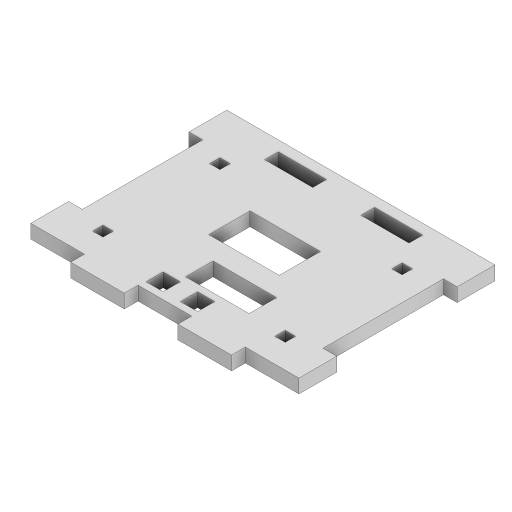
# Autodesk Inventor part: Front
Saved by Autodesk Inventor 2023.3 (Build 273359000, 359)
## iProperties
Created: 2024-06-25
Part Number: Front
Material: Generic
Document SubType Name: Modeling
Designer: David Zindović
Density: 1 g/cm^3
Appearance: Default
Author: David Zindović
Autodesk Inventor part; units mm, degrees
ref_plane "YZ Plane" through (0, 0, 0) normal (1, 0, 0) x (0, 1, 0)
ref_plane "XZ Plane" through (0, 0, 0) normal (0, 1, 0) x (-1, 0, 0)
ref_plane "XY Plane" through (0, 0, 0) normal (0, 0, 1) x (1, 0, 0)
sketch "Sketch1" plane through (0, 0, 0) normal (0, 1, 0) x (-1, 0, 0)
  line L0 (39, 23) -> (-39, 23)
  line L1 (-39, 23) -> (-39, -38)
  line L2 (-39, -38) -> (39, -38)
  line L3 (39, -38) -> (39, 23)
  line L4 (-7, -31) -> (-21, -31)
  line L5 (-21, -31) -> (-21, -35)
  line L6 (-21, -35) -> (-7, -35)
  line L7 (-7, -35) -> (-7, -31)
  line L8 (-39, 8) -> (-35, 8)
  line L9 (-35, 8) -> (-35, -27)
  line L10 (-35, -27) -> (-39, -27)
  line L11 (-39, -27) -> (-39, 8)
  line L12 (-7.8, 23) -> (-23.4, 23)
  line L13 (-23.4, 23) -> (-23.4, 19)
  line L14 (-23.4, 19) -> (-7.8, 19)
  line L15 (-7.8, 19) -> (-7.8, 23)
  line L16 (0, 0) -> (0, -17.5171)
  line L17 (7, -31) -> (21, -31)
  line L18 (21, -31) -> (21, -35)
  line L19 (21, -35) -> (7, -35)
  line L20 (7, -35) -> (7, -31)
  line L21 (39, 8) -> (35, 8)
  line L22 (35, 8) -> (35, -27)
  line L23 (35, -27) -> (39, -27)
  line L24 (23.4, 23) -> (23.4, 19)
  line L25 (23.4, 19) -> (7.8, 19)
  line L26 (7.8, 19) -> (7.8, 23)
  line L27 (-39, 19) -> (39, 19)
  point P0 (0, -38)
  point P1 (-39, -7.5)
  point P2 (-7, -33)
  point P3 (7, -33)
  point P4 (-7.8, 19)
  point P5 (-23.4, 19)
  point P6 (-39, -27)
  point P7 (39, -27)
  point P8 (39, 8)
  point P9 (23.4, 19)
  point P10 (7.8, 19)
  point P11 (35, -9.5)
  point P12 (-35, -9.5)
  dimension "d0" = 61
  dimension "d1" = 78
  dimension "d2" = 14
  dimension "d3" = 4
  dimension "d4" = 3
  dimension "d5" = 7
  dimension "d6" = 35
  dimension "d7" = 11
  dimension "d8" = 15.6
  dimension "d9" = 15.6
  dimension "d12" = 4
  dimension "d13" = 4
  dimension "d35" = 4
  constraints: 56 end point, 9 symmetric about line, 5 midpoint, 5 parallel, 4 horizontal, 4 horizontal alignment, 4 point on line, 3 perpendicular, 1 collinear, 1 vertical, 1 vertical alignment
  measures "d0" distance of L0.end L1.end
  measures "d1" distance of L1.end L2.end
  measures "d2" distance of L6.end L5.end
  measures "d3" distance of L5.end L4.end
  measures "d4" distance between parallel lines of L2 L6
  measures "d5" horizontal distance of L16.start point (-7, -33)
  measures "d6" distance of L8.end L9.end
  measures "d7" distance between parallel lines of L2 L10
  measures "d8" distance of L13.end L14.end
  measures "d9" distance between parallel lines of L1 L13
  measures "d12" distance of L9.end L10.end
  measures "d13" distance of L12.end L13.end
  measures "d35" distance of L22.end L23.end
extrude "Extrusion1" add sketch "Sketch1" along normal mid plane 4 contours L24 L25 L26 L0 | L3 L21 L22 L23 L2 L1 L10 L9 L8 L27 L14 L25 | L15 L14 L13 L0
sketch "Sketch2" plane through (0, 2, 0) normal (0, 1, 0) x (1, 0, 0)
  line L0 (35, 27) -> (39, 27) projected
  line L1 (35, 27) -> (15.5, 27) construction
  line L2 (15.5, -2) -> (-3, -2)
  line L3 (-3, -2) -> (-3, -10)
  line L4 (-3, -10) -> (15.5, -10)
  line L5 (15.5, -10) -> (15.5, -2)
  line L6 (21, 31) -> (7, 31) projected
  line L7 (7.5, -17) -> (2.5, -17)
  line L8 (2.5, -17) -> (2.5, -12)
  line L9 (2.5, -12) -> (7.5, -12)
  line L10 (7.5, -12) -> (7.5, -17)
  line L11 (0, 0) -> (0, -2.2371)
  line L12 (-7.5, -17) -> (-2.5, -17)
  line L13 (-2.5, -17) -> (-2.5, -12)
  line L14 (-2.5, -12) -> (-7.5, -12)
  line L15 (-7.5, -12) -> (-7.5, -17)
  line L16 (28, -12) -> (25, -12)
  line L17 (25, -12) -> (25, -9)
  line L18 (25, -9) -> (28, -9)
  line L19 (28, -9) -> (28, -12)
  line L20 (35, -8) -> (35, 27) projected
  line L21 (23.4, -19) -> (39, -19) projected
  line L22 (-28, -12) -> (-25, -12)
  line L23 (-25, -12) -> (-25, -9)
  line L24 (-25, -9) -> (-28, -9)
  line L25 (-28, -9) -> (-28, -12)
  line L26 (-10.25, 16) -> (10.25, 16)
  line L27 (10.25, 16) -> (10.25, 4)
  line L28 (10.25, 4) -> (-10.25, 4)
  line L29 (-10.25, 4) -> (-10.25, 16)
  line L30 (39, 38) -> (-39, 38) projected
  line L31 (7.8, -23) -> (23.4, -23) projected
  line L32 (28, 22) -> (25, 22)
  line L33 (25, 22) -> (25, 25)
  line L34 (25, 25) -> (28, 25)
  line L35 (28, 25) -> (28, 22)
  line L36 (-28, 22) -> (-25, 22)
  line L37 (-25, 22) -> (-25, 25)
  line L38 (-25, 25) -> (-28, 25)
  line L39 (-28, 25) -> (-28, 22)
  point P0 (14, 31)
  point P1 (5, -17)
  point P2 (-5, -17)
  point P3 (28, -10.5)
  point P4 (31.2, -19)
  point P5 (-28, -10.5)
  point P6 (0, 16)
  point P7 (0, 38)
  point P8 (26.5, 22)
  point P9 (26.5, -9)
  point P10 (-26.5, 22)
  dimension "d14" = 19.5
  dimension "d15" = 18.5
  dimension "d16" = 8
  dimension "d17" = 41
  dimension "d20" = 5
  dimension "d21" = 5
  dimension "d22" = 5
  dimension "d23" = 43
  dimension "d26" = 3
  dimension "d27" = 3
  dimension "d28" = 7
  dimension "d31" = 20.5
  dimension "d32" = 12
  dimension "d33" = 6
  dimension "d34" = 11
  dimension "d36" = 3
  dimension "d37" = 3
  dimension "d38" = 31
  constraints: 68 end point, 15 symmetric about line, 10 parallel, 8 midpoint, 6 horizontal, 5 perpendicular, 3 vertical alignment, 1 vertical
  measures "d14" distance of L0.start L1.end
  measures "d15" distance of L3.end L4.end
  measures "d16" distance of L2.end L3.end
  measures "d17" distance from line of point (14, 31) L4
  measures "d20" distance of L8.end L9.end
  measures "d21" distance of L7.end L8.end
  measures "d22" horizontal distance of L11.start point (5, -17)
  measures "d23" distance between parallel lines of L6 L9
  measures "d26" distance of L17.end L18.end
  measures "d27" distance of L16.end L17.end
  measures "d28" distance from line of L20 point (28, -10.5)
  measures "d31" distance of L27.end L28.end
  measures "d32" distance of L26.end L27.end
  measures "d33" distance between parallel lines of L28 L2
  measures "d34" distance between parallel lines of L16 L31
  measures "d36" distance of L33.end L34.end
  measures "d37" distance of L32.end L33.end
  measures "d38" distance between parallel lines of L32 L18
extrude "Extrusion2" cut sketch "Sketch2" against normal up to surface (4 mm away)
equation "\"d5\" = 0.5 * d2"
equation "\"d8\" = 0.2 * d1"
equation "\"d9\" = d8"
equation "\"d35\" = d12"
equation "\"d21\" = d20"
body "Solid1"
